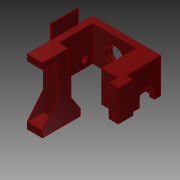
# Autodesk Inventor part: obudowa
Saved by Autodesk Inventor 2013 (Build 170138000, 138)
## iProperties
Created: 2014-04-23
Part Number: obudowa
Material: ABS Plastic
Document SubType Name: Modeling
Designer: Masta
Density: 1 g/cm^3
Author: Masta
Autodesk Inventor part; units mm, degrees
ref_plane "Work Plane10" through (0, 0, -20.3) normal (0, 0, -1) x (-1, 0, 0)
sketch "Sketch13" plane through (0, 0, -20.3) normal (0, 0, -1) x (-1, 0, 0)
  line L0 (-20.3, -18) -> (20.3, -18)
  line L1 (20.3, -18) -> (20.3, 18)
  line L2 (20.3, 18) -> (-20.3, 18)
  line L3 (-20.3, 18) -> (-20.3, -18)
  line L4 (-20.3, 11) -> (-27.8, 11)
  line L5 (-27.8, 11) -> (-27.8, 8.5)
  line L6 (-27.8, 8.5) -> (-20.3, 8.5)
  line L7 (-20.3, 11) -> (-20.3, 8.5)
  line L8 (20.3, 8.5) -> (20.3, 11)
  line L9 (20.3, 8.5) -> (27.8, 8.5)
  line L10 (27.8, 8.5) -> (27.8, 11)
  line L11 (27.8, 11) -> (20.3, 11)
  line L12 (18.3, 48.2) -> (18.3, 43.8)
  line L13 (2.3, 48.2) -> (2.3, 43.8)
  line L14 (2.6, 48.5) -> (18, 48.5)
  line L15 (18, 43.5) -> (2.6, 43.5)
  arc A0 (4.05, 37.5) -> (4.05, 42.2) centre (1.78875, 39.85) ccw
  arc A1 (16.55, 42.2) -> (16.55, 37.5) centre (18.81125, 39.85) ccw
  line L16 (20.3, 18) -> (27.8, 18)
  line L17 (27.8, 18) -> (27.8, 46)
  line L18 (27.8, 46) -> (-7.2, 46)
  line L19 (-7.2, 46) -> (-7.2, 18)
  line L20 (10.3, 48.5) -> (10.3, 18) construction
  line L21 (27.8, 11) -> (32.8, 11)
  line L22 (32.8, 11) -> (32.8, 51)
  line L23 (32.8, 51) -> (-22.2, 51)
  line L24 (-22.2, 51) -> (-22.2, 23)
  line L25 (-27.8, 11) -> (-27.8, 23)
  line L26 (-27.8, 23) -> (-22.2, 23)
  line L27 (-7.2, 18) -> (27.8, 18)
  line L28 (27.8, 18) -> (27.8, 18.6)
  line L29 (27.8, 18.6) -> (-7.2, 18.6)
  line L30 (-7.2, 18.6) -> (-7.2, 18)
  line L31 (-20.3, 11) -> (20.3, 11)
  line L32 (20.3, 11) -> (20.3, 11.6)
  line L33 (20.3, 11.6) -> (-20.3, 11.6)
  line L34 (-20.3, 11.6) -> (-20.3, 11)
  circle A2 centre (40.8, 47) radius 1.6
  circle A3 centre (-9.2, 47.85) radius 1.6
  circle A4 centre (-9.2, 31.85) radius 1.6
  circle A5 centre (40.8, 32.7) radius 1.6
  line L35 (19.3, 42.85) -> (19.3, 36.85)
  line L36 (19.3, 36.85) -> (1.3, 36.85)
  line L37 (1.3, 36.85) -> (1.3, 42.85)
  line L38 (1.3, 42.85) -> (19.3, 42.85)
  line L39 (-22.2, 28.7) -> (44.8, 28.7)
  line L40 (44.8, 28.7) -> (44.8, 51)
  line L41 (44.8, 51) -> (-22.2, 51)
  line L42 (-22.2, 51) -> (-22.2, 28.7)
  line L43 (44.8, 51) -> (44.2, 51)
  line L44 (44.2, 51) -> (44.2, 28.7)
  line L45 (44.2, 28.7) -> (44.8, 28.7)
  line L46 (44.8, 28.7) -> (44.8, 51)
  point P0 (0, 0)
  point P1 (2.3, 46)
  dimension "d71" = 15
  dimension "d73" = 5
  dimension "d74" = 5
  dimension "d75" = 5
  dimension "d125" = 0.6
  dimension "d126" = 0.6
  dimension "d127" = 0.6
  constraints: 50 end point, 11 parallel, 9 perpendicular, 6 point on line, 4 point on circle, 3 horizontal, 2 centre point, 2 midpoint, 2 vertical, 1 collinear, 13 other
  measures "d71" distance between parallel lines of L24 L19
  measures "d73" distance between parallel lines of L22 L17
  measures "d74" distance between parallel lines of L23 L18
  measures "d75" distance between parallel lines of L2 L26
  measures "d125" distance between parallel lines of L27 L29
  measures "d126" distance of L31.end L32.end
  measures "d127" distance of L40.end L43.end
ref_plane "Work Plane11" through (-20.3, -18, 0) normal (0, 0, 1) x (1, 0, 0)
sketch "Sketch13 outline for Extrusion11" plane through (0, 0, -20.3) normal (0, 0, -1) x (-1, 0, 0)
  line L0 (44.2, 51) -> (44.2, 28.7)
  line L1 (44.8, 51) -> (44.2, 51)
  line L2 (44.8, 28.7) -> (44.8, 51)
  line L3 (44.2, 28.7) -> (44.8, 28.7)
  line L4 (20.3, 18) -> (20.3, 11.6)
  line L5 (20.3, 11.6) -> (-20.3, 11.6)
  line L6 (-20.3, 11.6) -> (-20.3, 18)
  line L7 (-20.3, 18) -> (20.3, 18)
  line L8 (27.8, 46) -> (27.8, 18.6)
  line L9 (27.8, 18.6) -> (-7.2, 18.6)
  line L10 (-7.2, 18.6) -> (-7.2, 46)
  line L11 (-7.2, 46) -> (27.8, 46)
  line L12 (32.8, 11) -> (32.8, 51)
  line L13 (32.8, 51) -> (-22.2, 51)
  line L14 (-22.2, 51) -> (-22.2, 23)
  line L15 (-22.2, 23) -> (-27.8, 23)
  line L16 (-27.8, 23) -> (-27.8, 11)
  line L17 (-27.8, 11) -> (32.8, 11)
extrude "Extrusion11" add sketch "Sketch13 outline for Extrusion11" against normal up to surface (20.3 mm away)
sketch "Sketch14" plane through (-27.8, 46, -20.3) normal (0, -1, 0) x (1, 0, 0)
  circle A0 centre (17.5, 10.15) radius 8
  circle A1 centre (17.5, 10.15) radius 6
  line L0 (35, 0) -> (0, 0)
  line L1 (11.843146, 4.493146) -> (14.186292, 2.15)
  line L2 (14.186292, 2.15) -> (20.813708, 2.15)
  line L3 (20.813708, 2.15) -> (23.156854, 4.493146)
  line L4 (17.5, 10.15) -> (17.5, 2.15) construction
  point P0 (27.8, 20.3)
  point P1 (11.843146, 15.806854)
  point P2 (23.882538, 14.973195)
  dimension "d78" = 12
  dimension "d120" = 135
  constraints: 8 end point, 4 point on circle, 3 tangent, 1 centre point, 1 coincident, 1 midpoint, 1 parallel, 1 vertical
  measures "d78" diameter of A1
  measures "d120" angle of L3 L2
ref_plane "Work Plane12" through (-20.673366, 48.5, -20.523366) normal (0, 1, 0) x (-0.4584918, 0, 0.8886986)
sketch "Sketch14 outline for Extrusion12" plane through (-27.8, 46, -20.3) normal (0, -1, 0) x (1, 0, 0)
  arc A0 (23.156854, 4.493146) -> (11.843146, 4.493146) centre (17.5, 10.15) ccw
  line L0 (20.813708, 2.15) -> (23.156854, 4.493146)
  line L1 (14.186292, 2.15) -> (20.813708, 2.15)
  line L2 (11.843146, 4.493146) -> (14.186292, 2.15)
extrude "Extrusion12" cut sketch "Sketch14 outline for Extrusion12" against normal up to surface (2.5 mm away) draft 10
sketch "Sketch15" plane through (-10.3, 48.5, -10.15) normal (0, -1, 0) x (1, 0, 0)
  circle A0 centre (0, 0) radius 8.440817
  circle A1 centre (0, 0) radius 6.5
  line L0 (-3.496301, -8.440817) -> (3.496301, -8.440817)
  line L1 (-4.596194, -4.596194) -> (-2.692388, -6.5)
  line L2 (-2.692388, -6.5) -> (2.692388, -6.5)
  line L3 (2.692388, -6.5) -> (4.596194, -4.596194)
  point P0 (10.3, 10.15)
  point P1 (0, -6.5)
  dimension "d81" = 13
  dimension "d122" = 45
  constraints: 6 end point, 3 point on circle, 3 tangent, 1 centre point, 1 coincident, 1 midpoint, 1 parallel
  measures "d81" diameter of A1
  measures "d122" angle of L1 L2
extrude "Extrusion13" cut sketch "Sketch15" against normal up to next contours A1 | A1 L2 L1 | L3 L2 A1
sketch "Sketch16" plane through (0, 0, -20.3) normal (0, 0, -1) x (-1, 0, 0)
  line L0 (32.8, 11) -> (32.8, 51) projected
  line L1 (32.8, 51) -> (-22.2, 51) projected
  line L2 (-22.2, 51) -> (-22.2, 23) projected
  line L3 (-22.2, 23) -> (-27.8, 23) projected
  line L4 (-27.8, 23) -> (-27.8, 11) projected
  line L5 (-27.8, 11) -> (32.8, 11) projected
  line L6 (-7.2, 18.6) -> (-7.2, 46) projected
  line L7 (-7.2, 46) -> (27.8, 46) projected
  line L8 (27.8, 46) -> (27.8, 18.6) projected
  line L9 (27.8, 18) -> (20.3, 18) projected
  line L10 (20.3, 18) -> (-7.2, 18)
  line L11 (20.3, 11) -> (-20.3, 11)
  line L12 (44.2, 51) -> (44.2, 28.7) projected
  line L13 (27.8, 18) -> (27.8, 18.6)
  line L14 (-7.2, 18.6) -> (-7.2, 18)
  line L15 (44.8, 51) -> (44.2, 51) projected
  line L16 (-7.2, 18.6) -> (27.8, 18.6)
  point P0 (0, 0)
  constraints: 10 end point, 4 parallel, 1 collinear
extrude "Extrusion14" add sketch "Sketch16" along normal blind 3 contours L5 L4 L3 L2 L1 L0 | L16 L13 L9 L10 L14
sketch "Sketch17" plane through (22.2, 23, 0) normal (1, 0, 0) x (0, 0, -1)
  line L0 (0, 28) -> (23.3, 28)
  arc A0 (3.9, 14.5) -> (3.9, 19.2) centre (1.63875, 16.85) ccw
  arc A1 (16.4, 19.2) -> (16.4, 14.5) centre (18.66125, 16.85) ccw
  line L1 (1.63875, 16.85) -> (18.66125, 16.85) construction
  circle A2 centre (16.9, 16.85) radius 1.5
  circle A3 centre (16.9, 16.85) radius 2.5
  line L2 (18.15, 14.684936) -> (19.4, 15.406624)
  line L3 (19.4, 15.406624) -> (19.4, 18.293376)
  line L4 (19.4, 18.293376) -> (18.15, 19.015064)
  point P0 (0, -23)
  point P1 (19.4, 16.85)
  point P2 (20.3, 28)
  dimension "d86" = 3
  dimension "d88" = 5
  dimension "d124" = 60
  constraints: 8 end point, 7 point on circle, 4 centre point, 4 tangent, 1 coincident, 1 midpoint, 1 parallel, 1 point on line, 1 vertical, 8 other
  measures "d86" diameter of A2
  measures "d88" diameter of A3
  measures "d124" angle of L3 L4
extrude "Extrusion15" cut sketch "Sketch17" against normal up to surface (55 mm away) contours A2 | A3 | L3 L2 A3 | A3 L4 L3
ref_plane "Work Plane13" through (22.2, 39.85, -16.9) normal (0, 0, -1) x (-1, 0, 0)
sketch "Sketch18" plane through (22.2, 39.85, -16.9) normal (0, 0, -1) x (-1, 0, 0)
  line L0 (0, 0) -> (9.3, 0)
  line L1 (0, 6) -> (0, 0)
  line L2 (0, -6) -> (4, -6)
  line L3 (4, -6) -> (4, -8.25)
  line L4 (4, -8.25) -> (9.3, -8.25)
  line L5 (9.3, -8.25) -> (9.3, 0)
  line L6 (9.3, 8.25) -> (4, 8.25)
  line L7 (4, 8.25) -> (4, 6)
  line L8 (4, 6) -> (0, 6)
  line L9 (0, 0) -> (0, -6)
  line L10 (9.3, 0) -> (9.3, 8.25)
  point P0 (22.2, -39.85)
  dimension "d91" = 16.5
  dimension "d93" = 12
  dimension "d94" = 4
  dimension "d95" = 5.3
  constraints: 22 end point, 5 parallel, 5 perpendicular, 2 coincident, 2 collinear, 1 horizontal, 2 other
  measures "d91" distance between parallel lines of L4 L6
  measures "d93" distance between parallel lines of L2 L8
  measures "d94" distance of L7.end L1.start
  measures "d95" distance of L3.end L4.end
extrude "Extrusion16" cut sketch "Sketch18" along normal up to next
revolve "Revolution2" cut sketch "Sketch18" angle 360 about axis through (22.2, 39.85, -16.9) along (-1, 0, 0) contours L1 L8 L7 L6 L10 L0
sketch "Sketch19" plane through (-32.8, 11, 0) normal (0, -1, 0) x (1, 0, 0)
  circle A0 centre (8.5, -5.15) radius 2 projected
  circle A1 centre (8.5, -15.15) radius 2 projected
  circle A2 centre (57.1, -15.15) radius 2 projected
  circle A3 centre (57.1, -5.15) radius 2 projected
  line L0 (9.25, -5.9) -> (7.75, -5.9)
  line L1 (7.75, -5.9) -> (7.75, -4.4)
  line L2 (7.75, -4.4) -> (9.25, -4.4)
  line L3 (9.25, -4.4) -> (9.25, -5.9)
  line L4 (9.25, -5.9) -> (7.75, -4.4) construction
  line L5 (7.75, -5.9) -> (9.25, -4.4) construction
  point P0 (32.8, 0)
  dimension "d99" = 1.5
  dimension "d100" = 1.5
  constraints: 12 end point, 2 midpoint, 2 parallel, 1 horizontal, 1 perpendicular
  measures "d99" distance of L1.end L2.end
  measures "d100" distance of L0.end L1.end
extrude "Extrusion17" cut sketch "Sketch19" against normal up to surface (12 mm away) contours L0 L1 L2 L3
pattern_linear "Rectangular Pattern1" count 2 spacing 48.6 along (1, 0, 0) count 2 spacing 10 along (0, 0, -1) of "Extrusion17"
sketch "Sketch20" plane through (0, 0, -23.3) normal (0, 0, -1) x (-1, 0, 0)
  line L0 (32.8, 11) -> (32.8, 51) projected
  circle A0 centre (40.8, 47) radius 1.6 projected
  circle A1 centre (40.8, 32.7) radius 1.6 projected
  line L1 (1.3, 42.85) -> (19.3, 42.85) projected
  line L2 (19.3, 42.85) -> (19.3, 36.85) projected
  line L3 (19.3, 36.85) -> (1.3, 36.85) projected
  line L4 (-22.2, 28.7) -> (44.8, 28.7) projected
  line L5 (44.8, 28.7) -> (44.8, 51) projected
  line L6 (44.8, 51) -> (-22.2, 51) projected
  circle A2 centre (-9.2, 47.85) radius 1.6 projected
  circle A3 centre (-9.2, 31.85) radius 1.6 projected
  line L7 (32.8, 51) -> (44.8, 51)
  line L8 (44.8, 51) -> (44.8, 28.7)
  line L9 (44.8, 28.7) -> (32.8, 28.7)
  line L10 (32.8, 28.7) -> (32.8, 51)
  circle A4 centre (-9.2, 47.85) radius 1.6 projected
  circle A5 centre (-9.2, 31.85) radius 1.6 projected
  line L11 (1.3, 36.85) -> (1.3, 42.85) projected
  line L12 (-22.2, 51) -> (-22.2, 28.7) projected
  point P0 (0, 0)
  constraints: 8 end point, 2 parallel, 2 point on line, 1 horizontal, 1 perpendicular
extrude "Extrusion18" add sketch "Sketch20" against normal blind 4 contours L0 L6 L5 L4
sketch "Sketch21" plane through (0, 0, -23.3) normal (0, 0, -1) x (-1, 0, 0)
  circle A0 centre (-9.2, 47.85) radius 1.6 projected
  circle A1 centre (-9.2, 31.85) radius 1.6 projected
  point P0 (0, 0)
  constraints: 2 coincident
hole "Hole3" at (9.2, 47.85, -23.3) at (9.2, 31.85, -23.3) direction (0, 0, 1) diameter 1.5 depth 8 tip angle 118
sketch "Sketch22" plane through (0, 0, -23.3) normal (0, 0, -1) x (-1, 0, 0)
  line L0 (-22.2, 33.85) -> (-22.2, 23) projected
  line L1 (-22.2, 23) -> (-27.8, 23) projected
  line L2 (-27.8, 23) -> (-27.8, 11) projected
  line L3 (-27.8, 11) -> (32.8, 11) projected
  line L4 (32.8, 11) -> (32.8, 28.7) projected
  line L5 (27.8, 46) -> (27.8, 18.6) projected
  line L6 (27.8, 18.6) -> (-7.2, 18.6) projected
  line L7 (-7.2, 18.6) -> (-7.2, 46) projected
  line L8 (32.8, 28.7) -> (27.8, 28.7)
  line L9 (27.8, 28.7) -> (-7.2, 28.7) construction
  line L10 (-7.2, 28.7) -> (-22.2, 28.7)
  point P0 (0, 0)
  constraints: 6 end point, 3 point on line, 2 perpendicular, 1 collinear
extrude "Extrusion19" cut sketch "Sketch22" against normal blind 3
sketch "Sketch23" plane through (0, 0, -20.3) normal (0, 0, -1) x (-1, 0, 0)
  line L0 (-20.3, 18) -> (20.3, 18) projected
  line L1 (20.3, 11.6) -> (-20.3, 11.6) projected
  line L2 (32.8, 11) -> (-27.8, 11) projected
  line L3 (-7.2, 18.6) -> (27.8, 18.6) projected
  line L4 (-22.2, 23) -> (-22.2, 28.7) projected
  line L5 (20.3, 18) -> (20.3, 18.6)
  line L6 (20.3, 11.6) -> (20.3, 11)
  line L7 (-7.2, 18.6) -> (-7.2, 18)
  line L8 (-20.3, 11.6) -> (-20.3, 11)
  point P0 (0, 0)
  constraints: 8 end point, 4 point on line, 2 perpendicular, 1 collinear, 1 parallel
extrude "Extrusion20" cut sketch "Sketch23" against normal up to next
sketch "Sketch24" plane through (-32.8, 51, 0) normal (0, 0, 1) x (1, 0, 0)
  line L0 (12.5, -40) -> (12.5, -32.4) projected
  line L1 (5, -32.4) -> (12.5, -32.4) projected
  line L2 (5, -5) -> (5, -32.4) projected
  line L3 (40, -5) -> (5, -5) projected
  line L4 (40, -5) -> (40, -33) projected
  line L5 (53.1, -33) -> (40, -33) projected
  line L6 (53.1, -40) -> (53.1, -33) projected
  line L7 (60.6, -40) -> (53.1, -40) projected
  line L8 (60.6, -28) -> (60.6, -40) projected
  line L9 (55, -28) -> (60.6, -28) projected
  line L10 (55, 0) -> (55, -28) projected
  line L11 (0, 0) -> (55, 0) projected
  line L12 (0, -40) -> (0, 0) projected
  line L13 (12.5, -40) -> (0, -40) projected
  line L14 (-12, -22.3) -> (-12, 0) projected
  line L15 (-11.4, -22.3) -> (-12, -22.3) projected
  line L16 (-11.4, 0) -> (-11.4, -22.3) projected
  line L17 (-12, 0) -> (-11.4, 0) projected
  line L18 (12.5, -40) -> (0, -40)
  line L19 (0, -40) -> (0, -53)
  line L20 (0, -53) -> (12.5, -53)
  line L21 (12.5, -53) -> (12.5, -40)
  point P0 (32.8, -51)
  dimension "d134" = 13
  constraints: 8 end point, 2 parallel, 1 collinear, 1 horizontal, 1 perpendicular
  measures "d134" distance of L18.end L19.end
extrude "Extrusion21" add sketch "Sketch24" along normal blind 5
sketch "Sketch25" plane through (0, 0, -20.3) normal (0, 0, -1) x (-1, 0, 0)
  line L0 (20.3, 18.6) -> (20.3, 11) projected
  line L1 (32.8, 11) -> (20.3, 11) projected
  line L2 (32.8, 28.7) -> (32.8, 11) projected
  line L3 (27.8, 28.7) -> (32.8, 28.7) projected
  line L4 (27.8, 18.6) -> (27.8, 28.7) projected
  line L5 (20.3, 18.6) -> (27.8, 18.6) projected
  line L6 (20.3, 11) -> (32.8, 11) projected
  line L7 (20.3, -2) -> (20.3, 11) projected
  line L8 (32.8, -2) -> (20.3, -2) projected
  line L9 (32.8, 11) -> (32.8, -2) projected
  line L10 (20.3, 18.6) -> (27.8, 18.6)
  line L11 (27.8, 18.6) -> (27.8, 28.7)
  line L12 (27.8, 28.7) -> (20.3, 28.7)
  line L13 (20.3, 28.7) -> (20.3, 18.6)
  point P0 (0, 0)
  constraints: 8 end point, 2 parallel, 1 horizontal, 1 perpendicular
extrude "Extrusion22" add sketch "Sketch25" along normal blind 27.3
extrude "Extrusion23" cut sketch "Sketch25" along normal blind 22 contours L13 L12 L4 L5 | L1 L9 L8 L7
sketch "Sketch26" plane through (-20.3, -2, 0) normal (1, 0, 0) x (0, 0, -1)
  line L0 (42.3, 20.6) -> (-5, 20.6)
  line L1 (0, 13) -> (42.3, 13)
  line L2 (42.3, 13) -> (42.3, 0)
  line L3 (42.3, 30.7) -> (42.3, 20.6)
  line L4 (42.3, 30.7) -> (26.979893, 20.6)
  line L5 (26.115629, 13) -> (42.3, 0)
  point P0 (0, 2)
  constraints: 4 end point, 2 point on line
extrude "Extrusion24" add sketch "Sketch26" against normal blind 0.5
sketch "Sketch27" plane through (-32.8, 39.85, -16.9) normal (-1, 0, 0) x (0, 0, 1)
  line L0 (-25.4, -28.85) -> (-9.215629, -28.85)
  line L1 (-25.4, -41.85) -> (-25.4, -28.85)
  line L2 (-25.4, -41.85) -> (-9.215629, -28.85)
  point P0 (16.9, -39.85)
extrude "Extrusion25" add sketch "Sketch27" against normal blind 0.5
body "Solid2"
